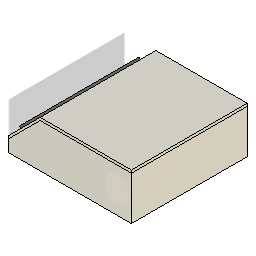
Hub v7 (Autodesk Fusion 360 design; units mm, degrees)
Autodesk Fusion 360 part; units mm, degrees
sketch "Sketch1" plane through (0, 0, 0) normal (0, 0, 1) x (1, 0, 0)
  line L0 (0, 0) -> (0, 90)
  line L1 (0, 90) -> (85, 90)
  line L2 (85, 90) -> (85, 0)
  line L3 (85, 0) -> (0, 0)
  dimension "d1" = 90
  dimension "d2" = 85
  constraint coincident L0.start L3.end
  constraint vertical L0
  constraint perpendicular L0 L1
  constraint perpendicular L1 L2
  constraint perpendicular L0 L3
  measures "d1" distance of L0.start L0.end
  measures "d2" distance of L0.end L1.end
extrude "Extrude1" add sketch "Sketch1" along normal blind 2 makes body 1
ref_plane "WorkPlane1" through (42.5, 45, 2) normal (0, 0, 1) x (1, 0, 0)
sketch "Sketch2" plane through (42.5, 45, 2) normal (0, 0, 1) x (1, 0, 0)
  line L0 (42.5, 45) -> (-42.5, 45)
  line L1 (-42.5, 45) -> (-42.5, -45)
  line L2 (-42.5, -45) -> (42.5, -45)
  line L3 (42.5, -45) -> (42.5, 45)
  line L4 (-40.5, -43) -> (40.5, -43)
  line L5 (40.5, -43) -> (40.5, 43)
  line L6 (40.5, 43) -> (-40.5, 43)
  line L7 (-40.5, 43) -> (-40.5, -43)
  dimension "d6" = 85
  dimension "d7" = 85
  dimension "d8" = -2
  constraint horizontal L0
  constraint perpendicular L0 L1
  constraint perpendicular L1 L2
  measures "d6" distance of L0.start L0.end
  measures "d7" distance of L1.end L2.end
extrude "Extrude2" add sketch "Sketch2" along normal blind 30 bodies 1
sketch "Sketch5" plane through (0, 0, 0) normal (0, 0, 1) x (1, 0, 0)
  line L0 (0, 0) -> (0, 35)
  line L1 (0, 35) -> (80, 35)
  line L2 (80, 35) -> (80, 0)
  line L3 (80, 0) -> (0, 0)
  dimension "d13" = 35
  dimension "d14" = 80
  constraint coincident L0.start L3.end
  constraint vertical L0
  constraint perpendicular L0 L1
  constraint perpendicular L1 L2
  constraint perpendicular L0 L3
  measures "d13" distance of L0.start L0.end
  measures "d14" distance of L0.end L1.end
extrude "Extrude4" add sketch "Sketch5" along normal blind 1 separate body makes body 2
sketch "Sketch6" plane through (0, 0, 1) normal (0, 0, 1) x (-1, 0, 0)
  line L0 (-80, 0) -> (-80, -35)
  line L1 (-80, -35) -> (0, -35)
  line L2 (0, -35) -> (0, 0)
  line L3 (0, 0) -> (-80, 0)
  line L4 (0, 0) -> (-80, 0)
  line L5 (-80, 0) -> (-80, -35)
  line L6 (-80, -35) -> (0, -35)
  line L7 (0, -35) -> (0, 0)
  line L8 (-75, -30) -> (-5, -30)
  line L9 (-5, -30) -> (-5, -5)
  line L10 (-5, -5) -> (-75, -5)
  line L11 (-75, -5) -> (-75, -30)
  dimension "d17" = -5
  constraint horizontal L4
  constraint vertical L5
  constraint horizontal L6
  constraint vertical L7
  constraint coincident L0.end L1.start
  constraint coincident L2.end L3.start
extrude "Extrude5" add sketch "Sketch6" along normal blind 8 contours L8 L9 L10 L11 bodies 2
sketch "Sketch7" plane through (0, 0, 9) normal (0, 0, 1) x (-1, 0, 0)
  line L0 (-75, -5) -> (-75, -30)
  line L1 (-75, -30) -> (-5, -30)
  line L2 (-5, -30) -> (-5, -5)
  line L3 (-5, -5) -> (-75, -5)
  line L4 (-75, -5) -> (-5, -5)
  line L5 (-5, -5) -> (-5, -30)
  line L6 (-5, -30) -> (-75, -30)
  line L7 (-75, -30) -> (-75, -5)
  line L8 (-9, -26) -> (-71, -26)
  line L9 (-71, -26) -> (-71, -9)
  line L10 (-71, -9) -> (-9, -9)
  line L11 (-9, -9) -> (-9, -26)
  dimension "d20" = 4
  constraint horizontal L4
  constraint vertical L5
  constraint horizontal L6
  constraint vertical L7
  constraint coincident L1.end L2.start
  constraint coincident L0.start L3.end
extrude "Extrude6" cut sketch "Sketch7" against normal blind 0.5 contours L8 L9 L10 L11 bodies 2
move_body "Move1" bodies 2 to x (1, 0, 0) y (0, 0.707107, 0.707107) z (0, -0.707107, 0.707107) at (2.5, 2, 2)
chamfer "Chamfer1" distance 23 angle 45 1 edges at (42.5, 0, 32) on bodies 1
move_body "Move2" bodies 2 to x (1, 0, 0) y (0, 1, 0) z (0, 0, 1) at (0, 0.15, 0)
move_body "Move3" bodies 2 to x (1, 0, 0) y (0, 1, 0) z (0, 0, 1) at (0, 0, 2.5)
move_body "Move4" bodies 2 to x (1, 0, 0) y (0, 1, 0) z (0, 0, 1) at (0, 0, 2)
move_body "Move5" bodies 2 to x (1, 0, 0) y (0, 1, 0) z (0, 0, 1) at (0, 1, -3)
ref_plane "WorkPlane5" through (0, 23, 0) normal (0, 1, 0) x (0, 0, 1)
sketch "Sketch12" plane through (0, 23, 0) normal (0, 1, 0) x (1, 0, 0)
  line L0 (0, -32) -> (0, -34)
  line L1 (0, -34) -> (85, -34)
  line L2 (85, -34) -> (85, -32)
  line L3 (85, -32) -> (0, -32)
  dimension "d39" = 2
  dimension "d40" = 85
  dimension "d41" = 85
  constraint vertical L0
  constraint perpendicular L0 L1
  constraint perpendicular L1 L2
  constraint perpendicular L2 L3
  measures "d39" distance of L0.start L0.end
  measures "d40" distance of L0.end L1.end
  measures "d41" distance of L2.end L0.start
sketch "Sketch13" plane through (0, 0, 0) normal (0, 1, 0) x (1, 0, 0)
  line L0 (0, -9) -> (0, -11)
  line L1 (0, -11) -> (85, -11)
  line L2 (85, -11) -> (85, -9)
  line L3 (85, -9) -> (0, -9)
  dimension "d42" = 85
  dimension "d43" = 85
  constraint vertical L0
  constraint perpendicular L0 L1
  constraint perpendicular L1 L2
  constraint perpendicular L2 L3
  measures "d42" distance of L0.end L1.end
  measures "d43" distance of L2.end L0.start
loft "Loft1" add profiles "Sketch12", "Sketch13" section 1 section 2 separate body makes body 3
extrude "Extrude8" add 1 faces at (28.3333, 23, 32.6667) along direction (0, 1, 0) blind 67 on bodies 3 bodies 3
hole "Hole1" at (80.353, 26.2691, 26.6191) direction (0, -0.707107, 0.707107) diameter 3 depth 3 tip angle 118 bodies 2
hole "Hole2" at (4.9487, 26.2352, 26.5852) direction (0, -0.707107, 0.707107) diameter 3 depth 3 tip angle 118 bodies 2
hole "Hole3" at (5.0421, 4.6196, 4.9696) direction (0, -0.707107, 0.707107) diameter 3 depth 3 tip angle 118 bodies 2
hole "Hole4" at (80.2872, 4.6614, 5.0114) direction (0, -0.707107, 0.707107) diameter 3 depth 3.5 tip angle 118 bodies 2
sketch "Sketch15" plane through (0, -5.5, 5.5) normal (0, -0.707107, 0.707107) x (1, 0, 0)
  line L0 (85, 40.3051) -> (0, 40.3051)
  line L1 (0, 40.3051) -> (0, 7.7782)
  line L2 (0, 7.7782) -> (85, 7.7782)
  line L3 (85, 7.7782) -> (85, 40.3051)
  line L4 (7.5, 34.7) -> (77.5, 34.7)
  line L5 (77.5, 34.7) -> (77.5, 9.7)
  line L6 (77.5, 9.7) -> (7.5, 9.7)
  line L7 (7.5, 9.7) -> (7.5, 34.7)
  constraint parallel L0 L4
  constraint perpendicular L4 L5
  constraint perpendicular L5 L6
extrude "Extrude9" cut sketch "Sketch15" against normal blind 2 contours L4 L5 L6 L7 bodies 3
sketch "Sketch18" plane through (0, -4.5, 4.5) normal (0, 0.707107, -0.707107) x (-1, 0, 0)
  line L0 (-77.5, 9.7) -> (-77.5, 34.7)
  line L1 (-77.5, 34.7) -> (-7.5, 34.7)
  line L2 (-7.5, 34.7) -> (-7.5, 9.7)
  line L3 (-7.5, 9.7) -> (-77.5, 9.7)
  line L4 (0, 38.8909) -> (-85, 38.8909)
  line L5 (-85, 38.8909) -> (-85, 6.364)
  line L6 (-85, 6.364) -> (0, 6.364)
  line L7 (0, 6.364) -> (0, 38.8909)
  circle A0 centre (-80.353, 37.3976) radius 1.5
  circle A1 centre (-80.353, 37.3976) radius 2
  circle A2 centre (-4.9487, 37.3497) radius 1.5
  circle A3 centre (-4.9487, 37.3497) radius 2
  circle A4 centre (-5.0421, 6.7806) radius 1.5
  circle A5 centre (-5.0421, 6.7806) radius 2
  circle A6 centre (-80.2872, 6.8397) radius 1.5
  circle A7 centre (-80.2872, 6.8397) radius 2
  circle A8 centre (-80.2872, 6.8397) radius 1
  circle A9 centre (-80.353, 37.3976) radius 1
  circle A10 centre (-4.9487, 37.3497) radius 1
  circle A11 centre (-5.0421, 6.7806) radius 1
  dimension "d61" = 3
  dimension "d62" = 4
  dimension "d63" = 3
  dimension "d64" = 4
  dimension "d65" = 3
  dimension "d66" = 4
  dimension "d67" = 3
  dimension "d68" = 4
  dimension "d69" = -1
  dimension "d70" = -1
  dimension "d71" = -1
  dimension "d72" = -1
  constraint concentric A0 A1
  constraint concentric A2 A3
  constraint concentric A4 A5
  constraint concentric A6 A7
  measures "d61" diameter of A0
  measures "d62" diameter of A1
  measures "d63" diameter of A2
  measures "d64" diameter of A3
  measures "d65" diameter of A4
  measures "d66" diameter of A5
  measures "d67" diameter of A6
  measures "d68" diameter of A7
extrude "Extrude10" add sketch "Sketch18" along normal blind 5 contours L6 A4 A11 | L6 A4 A11 | L4 A0 | L6 A6 A8 | L6 A6 A8 | A2 picked at (-80.3779, 38.7255) bodies 3
extrude "Extrude12" cut 2 faces at (81.4342, -0.1401, 8.8599) (6.2222, -0.1395, 8.8605) along direction (0, 0.707107, -0.707107) blind 1.2 on bodies 3 bodies 3
sketch "Sketch19" plane through (0, 0, 0) normal (0, 0, 1) x (1, 0, 0)
  line L0 (0, 0) -> (77, 0)
  line L1 (77, 0) -> (77, 21)
  line L2 (77, 21) -> (0, 21)
  line L3 (0, 21) -> (0, 0)
  dimension "d79" = 77
  dimension "d80" = 21
  dimension "d81" = 77
  constraint coincident L0.start L3.end
  constraint horizontal L0
  constraint perpendicular L0 L1
  constraint perpendicular L1 L2
  measures "d79" distance of L0.start L0.end
  measures "d80" distance of L0.end L1.end
  measures "d81" distance of L1.end L2.end
extrude "Extrude13" add sketch "Sketch19" along normal blind 1 separate body makes body 4
ref_plane "WorkPlane7" through (38.5, 10.5, 1) normal (0, 0, 1) x (1, 0, 0)
sketch "Sketch20" plane through (38.5, 10.5, 1) normal (0, 0, 1) x (1, 0, 0)
  line L0 (-38.5, 10.5) -> (-37.5, 10.5)
  line L1 (-37.5, 10.5) -> (-37.5, -10.5)
  line L2 (-37.5, -10.5) -> (-38.5, -10.5)
  line L3 (-38.5, -10.5) -> (-38.5, 10.5)
  line L4 (38.5, 10.5) -> (37.5, 10.5)
  line L5 (37.5, 10.5) -> (37.5, -10.5)
  line L6 (37.5, -10.5) -> (38.5, -10.5)
  line L7 (38.5, -10.5) -> (38.5, 10.5)
  line L8 (37.5, 10.5) -> (-37.5, 10.5)
  line L9 (-37.5, 10.5) -> (-37.5, 9.5)
  line L10 (-37.5, 9.5) -> (37.5, 9.5)
  line L11 (-37.5, -10.5) -> (-37.5, -9.5)
  line L12 (-37.5, -9.5) -> (37.5, -9.5)
  line L13 (37.5, -10.5) -> (-37.5, -10.5)
  dimension "d85" = 1
  dimension "d86" = 21
  dimension "d87" = 1
  dimension "d88" = 1
  dimension "d89" = 21
  dimension "d90" = 1
  dimension "d91" = 75
  dimension "d92" = 1
  dimension "d93" = 75
  constraint horizontal L0
  constraint perpendicular L0 L1
  constraint perpendicular L1 L2
  constraint horizontal L4
  constraint perpendicular L4 L5
  constraint perpendicular L5 L6
  constraint perpendicular L1 L8
  constraint perpendicular L0 L9
  constraint perpendicular L1 L10
  constraint perpendicular L2 L11
  constraint perpendicular L1 L12
  measures "d85" distance of L0.start L0.end
  measures "d86" distance of L0.end L1.end
  measures "d87" distance of L1.end L2.end
  measures "d88" distance of L4.start L4.end
  measures "d89" distance of L4.end L5.end
  measures "d90" distance of L0.end L9.end
  measures "d91" distance of L9.end L10.end
  measures "d92" distance of L1.end L11.end
  measures "d93" distance of L11.end L12.end
extrude "Extrude15" add sketch "Sketch20" along normal blind 10 contours L1 L5 L8 L9 L10 | L1 L5 L11 L12 L13 bodies 4
extrude "Extrude14" add sketch "Sketch20" along normal blind 20 contours L0 L1 L2 L3 L9 L11 | L4 L5 L6 L7 bodies 4
sketch "Sketch21" plane through (1, 0, 0) normal (1, 0, 0) x (0, 1, 0)
  line L0 (20, 11) -> (21, 11)
  line L1 (21, 11) -> (21, 21)
  line L2 (21, 21) -> (0, 21)
  line L3 (0, 21) -> (0, 11)
  line L4 (0, 11) -> (1, 11)
  line L5 (1, 11) -> (1, 1)
  line L6 (1, 1) -> (20, 1)
  line L7 (20, 1) -> (20, 11)
  circle A0 centre (10.5057, 10.5002) radius 9.1885
  dimension "d98" = 28.2843
  dimension "d99" = 28.2843
  measures "d98" distance of L2.end L6.end
  measures "d99" distance of L1.end L5.end
extrude "Extrude16" add sketch "Sketch21" along normal blind 75 contours A0 bodies 4
move_body "Move7" bodies 4 to x (1, 0, 0) y (0, 1, 0) z (0, 0, 1) at (4.5, 40, 0)
move_body "Move8" bodies 4 to x (1, 0, 0) y (0, 1, 0) z (0, 0, 1) at (0, 25, 20)
move_body "Move9" bodies 4 to x (1, 0, 0) y (0, 1, 0) z (0, 0, 1) at (0, 0, -18)
sketch "Sketch22" plane through (0, 0, 0) normal (0, 0, 1) x (1, 0, 0)
  line L0 (0, 0) -> (70, 0)
  line L1 (70, 0) -> (70, 50)
  line L2 (70, 50) -> (0, 50)
  line L3 (0, 50) -> (0, 0)
  dimension "d102" = 70
  dimension "d103" = 50
  constraint coincident L0.start L3.end
  constraint horizontal L0
  constraint perpendicular L0 L1
  constraint perpendicular L1 L2
  constraint perpendicular L0 L3
  measures "d102" distance of L0.start L0.end
  measures "d103" distance of L0.end L1.end
extrude "Extrude17" add sketch "Sketch22" along normal blind 1 separate body makes body 5
sketch "Sketch23" plane through (0, 0, 1) normal (0, 0, 1) x (-1, 0, 0)
  line L0 (0, -50) -> (0, 0)
  line L1 (0, 0) -> (-70, 0)
  line L2 (-70, 0) -> (-70, -50)
  line L3 (-70, -50) -> (0, -50)
  line L4 (0, 0) -> (-5, 0)
  line L5 (-5, 0) -> (-5, -50)
  line L6 (0, -50) -> (-5, -50)
  line L7 (0, -50) -> (0, 0)
  line L8 (-5, 0) -> (-8, 0)
  line L9 (-8, -50) -> (-5, -50)
  line L10 (-8, 0) -> (-8, -50)
  line L11 (-8, 0) -> (-35, 0)
  line L12 (-35, 0) -> (-35, -50)
  line L13 (-35, -50) -> (-38, -50)
  line L14 (-38, -50) -> (-38, 0)
  line L15 (-38, 0) -> (-35, 0)
  dimension "d106" = 5
  dimension "d107" = 27
  dimension "d108" = 3
  constraint coincident L0.end L1.start
  constraint perpendicular L0 L4
  constraint coincident L3 L5.end
  constraint perpendicular L3 L5
  constraint coincident L0.start L3.end
  constraint coincident L1 L8.end
  constraint perpendicular L5 L8
  constraint coincident L3 L9.start
  constraint perpendicular L9 L10
  constraint perpendicular L10 L11
  constraint midpoint L3 L12.end
  constraint coincident L3 L13.end
  constraint coincident L1 L14.end
  constraint perpendicular L1 L14
  constraint parallel L1 L15
  measures "d106" distance of L0.end L4.end
  measures "d107" distance of L8.end L11.end
  measures "d108" distance of L12.end L13.end
extrude "Extrude18" add sketch "Sketch23" along normal blind 3 contours L1 L3 L5 L8 L9 L10 | L1 L3 L12 L13 L14 L15 bodies 5
ref_plane "WorkPlane8" through (6.5, 25, 4) normal (0, 0, 1) x (1, 0, 0)
sketch "Sketch24" plane through (6.5, 25, 4) normal (0, 0, 1) x (1, 0, 0)
  line L0 (-1.5, 25) -> (31.5, 25)
  line L1 (31.5, 25) -> (31.5, -32)
  line L2 (31.5, -32) -> (-1.5, -32)
  line L3 (-1.5, -32) -> (-1.5, 25)
  dimension "d112" = 57
  constraint horizontal L0
  constraint perpendicular L0 L1
  constraint perpendicular L1 L2
  measures "d112" distance of L0.end L1.end
extrude "Extrude19" add sketch "Sketch24" along normal blind 1 bodies 5
move_body "Move10" bodies 5 to x (1, 0, 0) y (0, 1, 0) z (0, 0, 1) at (0, 15, 2)
move_body "Move11" bodies 5 to x (1, 0, 0) y (0, 1, 0) z (0, 0, 1) at (0, 0, 7)
extrude "Extrude20" cut 1 faces at (70, 31.6667, 9.6667) along direction (-1, 0, 0) blind 31 on bodies 5 bodies 5
move_body "Move12" bodies 5 to x (0, 1, 0) y (-1, 0, 0) z (0, 0, 1) at (67.6163, 25.5417, 0)
sketch "Sketch25" plane through (0, 0, 0) normal (0, 0, 1) x (1, 0, 0)
  line L0 (0, 0) -> (28, 0)
  line L1 (28, 0) -> (28, 17.3)
  line L2 (28, 17.3) -> (0, 17.3)
  line L3 (0, 17.3) -> (0, 0)
  dimension "d117" = 28
  dimension "d118" = 17.3
  constraint coincident L0.start L3.end
  constraint horizontal L0
  constraint perpendicular L0 L1
  constraint perpendicular L1 L2
  constraint perpendicular L0 L3
  measures "d117" distance of L0.start L0.end
  measures "d118" distance of L0.end L1.end
extrude "Extrude21" add sketch "Sketch25" along normal blind 1 separate body makes body 6
sketch "Sketch26" plane through (0, 0, 1) normal (0, 0, 1) x (-1, 0, 0)
  line L0 (0, -17.3) -> (0, 0)
  line L1 (0, 0) -> (-28, 0)
  line L2 (-28, 0) -> (-28, -17.3)
  line L3 (-28, -17.3) -> (0, -17.3)
  line L4 (1, -12.5) -> (-4, -12.5)
  line L5 (-4, -12.5) -> (-4, -10.5)
  line L6 (-4, -10.5) -> (1, -10.5)
  line L7 (1, -10.5) -> (1, -12.5)
  constraint horizontal L4
  constraint vertical L5
  constraint horizontal L6
  constraint vertical L7
extrude "Extrude22" add sketch "Sketch26" along normal blind 3 contours L0 L4 L5 L6 | L0 L4 L6 L7 bodies 6
extrude "Extrude23" add 1 faces at (1, 10.5, 3) along direction (0, -1, 0) blind 6 on bodies 6 bodies 6
extrude "Extrude24" cut 1 faces at (1, 12.5, 3) along direction (0, -1, 0) blind 3 on bodies 6 bodies 6
move_body "Move13" bodies 6 to x (-1, 0, 0) y (0, -1, 0) z (0, 0, 1) at (53, 25, 2)
move_body "Move14" bodies 6 to x (1, 0, 0) y (0, 1, 0) z (0, 0, 1) at (30, 32, 0)
named bodies: "нижний короб", "экрат", "врехний короб", "аккумулятор", "ESP 8266", "плата зарядки"
